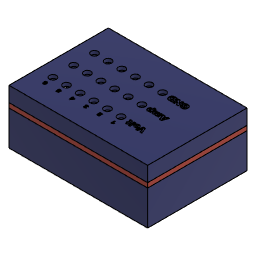
ESP-Messbox v10 (Autodesk Fusion 360 design; units mm, degrees)
Autodesk Fusion 360 part; units mm, degrees
sketch "Skizze1" plane through (0, 0, 0) normal (0, 0, 1) x (1, 0, 0) in component "BoxUnten"
  line L0 (0, 0) -> (116, 0)
  line L1 (116, 0) -> (116, 82)
  line L2 (116, 82) -> (0, 82)
  line L3 (0, 82) -> (0, 0)
  line L4 (-2, -2) -> (118, -2)
  line L5 (118, -2) -> (118, 84)
  line L6 (118, 84) -> (-2, 84)
  line L7 (-2, 84) -> (-2, -2)
  circle A0 centre (8, 76) radius 3
  circle A1 centre (108, 76) radius 3
  circle A2 centre (8, 7) radius 3
  circle A3 centre (108, 7) radius 3
  circle A4 centre (8, 76) radius 4
  circle A5 centre (108, 76) radius 4
  circle A6 centre (8, 7) radius 4
  circle A7 centre (108, 7) radius 4
  circle A8 centre (8, 76) radius 1.25
  circle A9 centre (108, 76) radius 1.25
  circle A10 centre (108, 7) radius 1.25
  circle A11 centre (8, 7) radius 1.25
  dimension "d1" = 116
  dimension "d2" = 82
  dimension "d4" = 2
  dimension "d10" = 6
  dimension "d11" = 1
  dimension "d12" = 1
  dimension "d13" = 1
  dimension "d14" = 1
  dimension "d32" = 100
  dimension "d33" = 8
  dimension "d34" = 69
  dimension "d35" = 6
  dimension "d36" = 2.5
  constraint horizontal L0
  constraint vertical L1
  constraint horizontal L2
  constraint vertical L3
  constraint coincident L0.start L3.end
  constraint equal A0 A2
  constraint equal A0 A3
  constraint equal A0 A1
  constraint horizontal A0.centre A1.centre
  constraint vertical A0.centre A2.centre
  constraint horizontal A2.centre A3.centre
  constraint vertical A1.centre A3.centre
  constraint concentric A0 A8
  constraint concentric A1 A9
  constraint concentric A3 A10
  constraint concentric A2 A11
  constraint equal A8 A9
  constraint equal A8 A11
  constraint equal A8 A10
  measures "d1" distance of L1.end L2.end
  measures "d2" distance of L0.end L1.end
  measures "d10" diameter of A0
  measures "d32" distance of A0.centre A1.centre
  measures "d33" horizontal distance of L2.end A0.centre
  measures "d34" distance of A0.centre A2.centre
  measures "d35" vertical distance of L2.end A0.centre
  measures "d36" diameter of A8
extrude "Extrusion1" add sketch "Skizze1" along normal blind 30 contours L4 L5 L6 L7 makes body 1 in component "BoxUnten"
extrude "Extrusion2" add sketch "Skizze1" along normal blind 2.5 contours L0 L1 L2 L3 | A0 | A1 | A2 | A3 | A4 | A5 | A6 | A7 | A8 | A9 | A10 | A11 bodies 1 in component "BoxUnten"
extrude "Extrusion3" add sketch "Skizze1" along normal blind 5 contours A0 | A1 | A2 | A3 | A4 | A5 | A6 | A7 | A8 | A9 | A10 | A11 bodies 1 in component "BoxUnten"
extrude "Extrusion4" add sketch "Skizze1" along normal blind 7 contours A0 | A1 | A2 | A3 | A8 | A9 | A10 | A11 bodies 1 in component "BoxUnten"
sketch "Skizze2" plane through (-2, 0, 0) normal (-1, 0, 0) x (0, -1, 0) in component "BoxUnten"
  line L0 (-84, 0) -> (2, 0)
  line L1 (2, 0) -> (2, 30)
  line L2 (2, 30) -> (-84, 30)
  line L3 (-84, 30) -> (-84, 0)
  circle A0 centre (-44, 22) radius 4.1
  circle A1 centre (-34, 22) radius 2.5
  dimension "d19" = 8.2
  dimension "d20" = 5
  dimension "d21" = 40
  dimension "d22" = 22
  dimension "d23" = 10
  constraint horizontal A0.centre A1.centre
  measures "d19" diameter of A0
  measures "d20" diameter of A1
  measures "d21" horizontal distance of L0.start A0.centre
  measures "d22" vertical distance of L0.start A0.centre
  measures "d23" distance of A0.centre A1.centre
sketch "Skizze3" plane through (0, 0, 30) normal (0, 0, 1) x (-1, 0, 0) in component "BoxUnten"
  line L0 (0, 0) -> (0, -82)
  line L1 (0, -82) -> (-116, -82)
  line L2 (-116, -82) -> (-116, 0)
  line L3 (-116, 0) -> (0, 0)
  line L4 (2, -84) -> (2, 2)
  line L5 (2, 2) -> (-118, 2)
  line L6 (-118, 2) -> (-118, -84)
  line L7 (-118, -84) -> (2, -84)
  circle A0 centre (-108, -76) radius 4
  circle A1 centre (-8, -76) radius 4
  circle A2 centre (-108, -7) radius 4
  circle A3 centre (-8, -7) radius 4
  line L8 (0, -82) -> (0, 0)
  line L9 (0, 0) -> (-116, 0)
  line L10 (-116, 0) -> (-116, -82)
  line L11 (-116, -82) -> (0, -82)
  line L12 (-114.5, -1.5) -> (-1.5, -1.5)
  line L13 (-1.5, -1.5) -> (-1.5, -80.5)
  line L14 (-1.5, -80.5) -> (-114.5, -80.5)
  line L15 (-114.5, -80.5) -> (-114.5, -1.5)
  dimension "d26" = 1.5
extrude "Extrusion6" add sketch "Skizze3" along normal blind 10 and the other way blind 12 contours L0 L1 L2 L3 L8 L9 L10 L11 bodies 1 in component "BoxUnten"
extrude "Extrusion5" cut sketch "Skizze2" against normal up to surface (3.5 mm away) contours A0 | A1 bodies 1 in component "BoxUnten"
sketch "Skizze1 (2)" plane through (0, 0, 7) normal (0, 0, 1) x (-1, 0, 0)
  circle A0 centre (-8, -76) radius 3
  circle A1 centre (-8, -7) radius 1.25
  circle A2 centre (-8, -76) radius 1.25
  circle A3 centre (-108, -7) radius 1.25
  circle A4 centre (-108, -76) radius 1.25
extrude "Extrusion7" cut sketch "Skizze1 (2)" against normal blind 4 contours A1 | A2 | A3 | A4 bodies 1 in component "BoxUnten"
fillet "Abrundung1" radius 1 4 edges at (5.203, 74.9152, 7) (105.203, 74.9152, 7) (5.203, 5.9152, 7) (105.203, 5.9152, 7) on bodies 1 in component "BoxUnten"
sketch "Skizze1 (3)" plane through (0, 0, 30) normal (0, 0, 1) x (-1, 0, 0) in component "BoxOben"
  line L0 (0, 0) -> (0, -82)
  line L1 (0, -82) -> (-116, -82)
  line L2 (-116, -82) -> (-116, 0)
  line L3 (-116, 0) -> (0, 0)
  line L4 (2, -84) -> (2, 2)
  line L5 (2, 2) -> (-118, 2)
  line L6 (-118, 2) -> (-118, -84)
  line L7 (-118, -84) -> (2, -84)
  line L8 (2, -84) -> (2, 2)
  line L9 (-118, -84) -> (2, -84)
  line L10 (-118, 2) -> (-118, -84)
  line L11 (2, 2) -> (-118, 2)
  line L12 (-1.5, -80.5) -> (-114.5, -80.5)
  line L13 (-114.5, -80.5) -> (-114.5, -1.5)
  line L14 (-114.5, -1.5) -> (-1.5, -1.5)
  line L15 (-1.5, -1.5) -> (-1.5, -80.5)
  line L16 (-116, -82) -> (0, -82)
  line L17 (0, -82) -> (0, 0)
  line L18 (0, 0) -> (-116, 0)
  line L19 (-116, 0) -> (-116, -82)
extrude "Extrusion1'" add sketch "Skizze1 (3)" along normal blind 14 separate body contours L4 L5 L6 L7 L8 L9 L10 L11 makes body 2 in component "BoxOben"
sketch "Skizze2 (2)" plane through (0, 0, 40) normal (0, 0, 1) x (-1, 0, 0) in component "BoxOben"
  line L0 (-1.5, -80.5) -> (-114.5, -80.5)
  line L1 (-114.5, -80.5) -> (-114.5, -1.5)
  line L2 (-114.5, -1.5) -> (-1.5, -1.5)
  line L3 (-1.5, -1.5) -> (-1.5, -80.5)
  line L4 (-116, -82) -> (0, -82)
  line L5 (0, -82) -> (0, 0)
  line L6 (0, 0) -> (-116, 0)
  line L7 (-116, 0) -> (-116, -82)
extrude "Extrusion2'" add sketch "Skizze2 (2)" along normal up to surface (4 mm away) bodies 2 in component "BoxOben"
sketch "Skizze3 (2)" plane through (0, 0, 44) normal (0, 0, 1) x (-1, 0, 0) in component "BoxOben"
  line L0 (-114.5, -80.5) -> (-114.5, -1.5)
  line L1 (-114.5, -1.5) -> (-1.5, -1.5)
  line L2 (-1.5, -1.5) -> (-1.5, -80.5)
  line L3 (-1.5, -80.5) -> (-114.5, -80.5)
  line L4 (2, 2) -> (-118, 2)
  line L5 (-118, 2) -> (-118, -84)
  line L6 (-118, -84) -> (2, -84)
  line L7 (2, -84) -> (2, 2)
  line L8 (2, 2) -> (-118, 2)
  line L9 (-118, 2) -> (-118, -84)
  line L10 (2, -84) -> (2, 2)
  line L11 (-118, -84) -> (2, -84)
  line L12 (-118, -41) -> (2, -41) construction
  line L13 (-58, 2) -> (-58, -84) construction
  circle A0 centre (-70, -41) radius 3
  circle A1 centre (-70, -59) radius 3
  circle A2 centre (-58.2, -59) radius 3
  circle A3 centre (-46.4, -59) radius 3
  circle A4 centre (-34.6, -59) radius 3
  circle A5 centre (-22.8, -59) radius 3
  circle A6 centre (-11, -59) radius 3
  circle A7 centre (-58.2, -41) radius 3
  circle A8 centre (-46.4, -41) radius 3
  circle A9 centre (-34.6, -41) radius 3
  circle A10 centre (-22.8, -41) radius 3
  circle A11 centre (-11, -41) radius 3
  circle A12 centre (-70, -23) radius 3
  circle A13 centre (-58.2, -23) radius 3
  circle A14 centre (-46.4, -23) radius 3
  circle A15 centre (-34.6, -23) radius 3
  circle A16 centre (-22.8, -23) radius 3
  circle A17 centre (-11, -23) radius 3
  dimension "d47" = 6
  dimension "d49" = 12
  dimension "d52" = 59
  dimension "d53" = 18
  constraint midpoint L9 L12.start
  constraint midpoint L10 L12.end
  constraint midpoint L4 L13.start
  constraint midpoint L6 L13.end
  constraint coincident L12 A0.centre
  measures "d47" diameter of A0
  measures "d49" distance of L13 A0.centre
extrude "Extrusion3'" add sketch "Skizze3 (2)" along normal blind 3 contours L0 L1 L2 L3 | L4 L5 L6 L7 L8 L9 L10 L11 bodies 2 in component "BoxOben"
sketch "Skizze4" plane through (0, 0, 47) normal (0, 0, 1) x (-1, 0, 0) in component "BoxOben"
  circle A0 centre (-22.8, -23) radius 3
  circle A1 centre (-58.2, -23) radius 3
  circle A2 centre (-58.2, -41) radius 3
  circle A3 centre (-34.6, -59) radius 3
  circle A4 centre (-11, -59) radius 3
  circle A5 centre (-34.6, -41) radius 3
  circle A6 centre (-46.4, -41) radius 3
  circle A7 centre (-46.4, -23) radius 3
  circle A8 centre (-58.2, -59) radius 3
  circle A9 centre (-22.8, -59) radius 3
  circle A10 centre (-46.4, -59) radius 3
  circle A11 centre (-70, -23) radius 3
  circle A12 centre (-11, -41) radius 3
  circle A13 centre (-22.8, -41) radius 3
  circle A14 centre (-70, -59) radius 3
  circle A15 centre (-11, -23) radius 3
  circle A16 centre (-34.6, -23) radius 3
  circle A17 centre (-70, -41) radius 3
  line L0 (-118, -84) -> (2, -84)
  line L1 (2, -84) -> (2, 2)
  line L2 (2, 2) -> (-118, 2)
  line L3 (-118, 2) -> (-118, -84)
  line L4 (-92.492, -61.1852) -> (-75.4195, -61.543) construction
  line L5 (-75.4195, -61.543) -> (-75.3072, -56.1832) construction
  line L6 (-75.3072, -56.1832) -> (-92.3796, -55.8254) construction
  line L7 (-92.3796, -55.8254) -> (-92.492, -61.1852) construction
  line L8 (-92.1166, -44.0076) -> (-75, -44) construction
  line L9 (-75, -44) -> (-75.0028, -37.6631) construction
  line L10 (-75.0028, -37.6631) -> (-92.1194, -37.6707) construction
  line L11 (-92.1194, -37.6707) -> (-92.1166, -44.0076) construction
  line L12 (-91.1792, -26.0263) -> (-75, -26) construction
  line L13 (-75, -26) -> (-75.0101, -19.7843) construction
  line L14 (-75.0101, -19.7843) -> (-91.1893, -19.8107) construction
  line L15 (-91.1893, -19.8107) -> (-91.1792, -26.0263) construction
  line L16 (-72, -19) -> (-68, -19) construction
  line L17 (-68, -19) -> (-68, -14) construction
  line L18 (-68, -14) -> (-72, -14) construction
  line L19 (-72, -14) -> (-72, -19) construction
  line L20 (-60.2, -19) -> (-56.2, -19) construction
  line L21 (-56.2, -19) -> (-56.2, -14) construction
  line L22 (-56.2, -14) -> (-60.2, -14) construction
  line L23 (-60.2, -14) -> (-60.2, -19) construction
  line L24 (-48.4, -19) -> (-44.4, -19) construction
  line L25 (-44.4, -19) -> (-44.4, -14) construction
  line L26 (-44.4, -14) -> (-48.4, -14) construction
  line L27 (-48.4, -14) -> (-48.4, -19) construction
  line L28 (-36.6, -19) -> (-32.6, -19) construction
  line L29 (-32.6, -19) -> (-32.6, -14) construction
  line L30 (-32.6, -14) -> (-36.6, -14) construction
  line L31 (-36.6, -14) -> (-36.6, -19) construction
  line L32 (-24.8, -19) -> (-20.8, -19) construction
  line L33 (-20.8, -19) -> (-20.8, -14) construction
  line L34 (-20.8, -14) -> (-24.8, -14) construction
  line L35 (-24.8, -14) -> (-24.8, -19) construction
  line L36 (-13, -19) -> (-9, -19) construction
  line L37 (-9, -19) -> (-9, -14) construction
  line L38 (-9, -14) -> (-13, -14) construction
  line L39 (-13, -14) -> (-13, -19) construction
  line L40 (-72, -14) -> (-9, -14) construction
  dimension "d54" = 5
  dimension "d55" = 5
  dimension "d56" = 5
  dimension "d64" = 3
  dimension "d65" = 3
  dimension "d66" = 3
  dimension "d67" = 3
  dimension "d68" = 3
  dimension "d69" = 3
  dimension "d74" = 4
  dimension "d75" = 4
  dimension "d76" = 4
  dimension "d77" = 4
  dimension "d78" = 4
  dimension "d79" = 5
  dimension "d80" = 4
  dimension "d81" = 9
  text T0 "GND" font "Arial Black" height 5 align left top in box 17.0762 x 5.361 at (-92.492, -61.1852) x (0.99978, -0.020952) y (0.020952, 0.99978) spacing 1 kerned
  text T1 "Amp" font "Arial Black" height 5 align left top in box 17.1166 x 6.3369 at (-92.1166, -44.0076) x (1, 0.000444) y (-0.000444, 1) spacing 1 kerned
  text T2 "Volt" font "Arial Black" height 5 align left top in box 16.1793 x 6.2157 at (-91.1792, -26.0263) x (0.999999, 0.001627) y (-0.001627, 0.999999) spacing 1 kerned
  text T3 "1\n" font "Arial Black" height 3 align left top in box 4 x 5 at (-72, -19) x (1, 0) y (0, 1) spacing 1 kerned
  text T4 "2\n" font "Arial Black" height 3 align left top in box 4 x 5 at (-60.2, -19) x (1, 0) y (0, 1) spacing 1 kerned
  text T5 "3" font "Arial Black" height 3 align left top in box 4 x 5 at (-48.4, -19) x (1, 0) y (0, 1) spacing 1 kerned
  text T6 "4\n" font "Arial Black" height 3 align left top in box 4 x 5 at (-36.6, -19) x (1, 0) y (0, 1) spacing 1 kerned
  text T7 "5\n" font "Arial Black" height 3 align left top in box 4 x 5 at (-24.8, -19) x (1, 0) y (0, 1) spacing 1 kerned
  text T8 "6\n" font "Arial Black" height 3 align left top in box 4 x 5 at (-13, -19) x (1, 0) y (0, 1) spacing 1 kerned
  constraint vertical A1.centre
  constraint vertical A7.centre
  constraint vertical A16.centre
  constraint vertical A0.centre
  constraint vertical A15.centre
  constraint vertical A11.centre
  constraint horizontal L40
  constraint coincident L40
  constraint coincident L18.end
  constraint coincident L37.end
  measures "d79" distance of L18.end
  measures "d81" distance of A11.centre
extrude "Extrusion4'" cut sketch "Skizze4" against normal blind 0.5 text T2 T1 T0 T3 T4 T5 T6 T7 T8 bodies 2 in component "BoxOben"
sketch "Skizze1 (4)" plane through (0, 0, 30) normal (0, 0, 1) x (-1, 0, 0) in component "Einleger"
  line L0 (0, 0) -> (0, -82)
  line L1 (0, -82) -> (-116, -82)
  line L2 (-116, -82) -> (-116, 0)
  line L3 (-116, 0) -> (0, 0)
  line L4 (2, -84) -> (2, 2)
  line L5 (2, 2) -> (-118, 2)
  line L6 (-118, 2) -> (-118, -84)
  line L7 (-118, -84) -> (2, -84)
extrude "Extrusion1''" add sketch "Skizze1 (4)" along normal blind 4 separate body makes body 3 in component "Einleger"
component "BoxUnten" placed x (1, 0, 0) y (0, 1, 0) z (0, 0, 1) at (0, 0, 0)
component "BoxOben" placed x (1, 0, 0) y (0, 1, 0) z (0, 0, 1) at (0, 0, 0)
component "Einleger" placed x (1, 0, 0) y (0, 1, 0) z (0, 0, 1) at (0, 0, 0)
